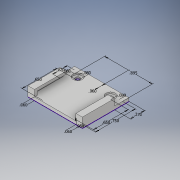
# Autodesk Inventor part: ShockSensorMount
Saved by Autodesk Inventor 2017 (Build 210142000, 142)
## iProperties
Created: 2018-12-12
Part Number: ShockSensorMount
Material: Glass
Document SubType Name: Modeling
Designer: S346795925
Density: 2.18 g/cm^3
Appearance: Clear
Author: S346795925
Autodesk Inventor part; units mm, degrees
sketch "Sketch1" plane through (0, 0, 0) normal (0, 1, 0) x (-1, 0, 0)
  line L0 (0, 0) -> (-25.781, 0)
  line L1 (-25.781, 0) -> (-25.781, -22.098)
  line L2 (-25.781, -22.098) -> (0, -22.098)
  line L3 (0, -22.098) -> (0, 0)
  line L4 (-1.524, -20.574) -> (-24.257, -20.574)
  line L5 (-24.257, -20.574) -> (-24.257, -1.524)
  line L6 (-24.257, -1.524) -> (-1.524, -1.524)
  line L7 (-1.524, -1.524) -> (-1.524, -20.574)
  line L8 (-3.048, 0) -> (-3.048, -1.524)
  line L9 (-22.733, 0) -> (-22.733, -1.524)
  line L10 (-3.048, -20.574) -> (-3.048, -22.098)
  line L11 (-3.048, -1.524) -> (-3.048, -20.574)
  line L12 (-22.733, -1.524) -> (-22.733, -20.574)
  line L13 (-22.733, -20.574) -> (-22.733, -22.098)
  line L14 (0, -15.24) -> (-1.524, -15.24)
  line L15 (-24.257, -15.24) -> (-25.781, -15.24)
  line L16 (-1.524, -15.24) -> (-3.048, -15.24)
  line L17 (-24.257, -15.24) -> (-22.733, -15.24)
  circle A0 centre (-5.08, -18.542) radius 1.0668
  circle A1 centre (-20.701, -2.032) radius 1.0668
  circle A2 centre (-20.701, -18.542) radius 1.0668
  circle A3 centre (-5.08, -2.032) radius 1.0668
  dimension "d2" = 1.524
  dimension "d3" = 19.05
  dimension "d4" = 22.733
  dimension "d5" = 1.524
  dimension "d6" = 1.524
  dimension "d10" = 6.858
  dimension "d11" = 6.858
  dimension "d19" = 2.1336
  dimension "d22" = 2.032
  dimension "d23" = 2.032
  dimension "d24" = 2.032
  dimension "d25" = 16.51
  dimension "d26" = 16.51
  constraints: 36 end point, 14 point on line, 12 perpendicular, 4 centre point, 4 parallel, 3 equal radius, 2 vertical alignment, 1 horizontal, 1 horizontal alignment, 3 other
  measures "d2" distance between parallel lines of L2 L4
  measures "d3" distance of L4.end L5.end
  measures "d4" distance of L4.start L4.end
  measures "d5" distance between parallel lines of L7 L8
  measures "d6" distance between parallel lines of L5 L9
  measures "d10" distance between parallel lines of L2 L14
  measures "d11" distance between parallel lines of L2 L15
  measures "d19" diameter of A1
  measures "d22" distance from line of L4 A0.centre
  measures "d23" distance from line of L11 A0.centre
  measures "d24" distance from line of L12 A2.centre
  measures "d25" distance of A3.centre A0.centre
  measures "d26" distance of A1.centre A2.centre
extrude "Extrusion2" add sketch "Sketch1" along normal blind 3.302 contours L3 L14 L7 L6 L8 L0 | L9 L6 L5 L15 L1 L0
ref_plane "Work Plane1" through (0, 3.302, 0) normal (0, 1, 0) x (1, 0, 0)
ref_plane "Work Plane2" through (0, 4.572, 0) normal (0, 1, 0) x (1, 0, 0)
extrude "Extrusion3" add sketch "Sketch1" along normal up to surface (1.27 mm away) from surface at 3.302 contours L3 L14 L7 L6 L8 L0 | L9 L6 L5 L15 L1 L0 | L6 L7 L16 L11 | L12 L17 L5 L6
ref_plane "Work Plane3" through (0, 1.524, 0) normal (0, 1, 0) x (1, 0, 0)
sketch "Sketch2" plane through (0, 1.524, 0) normal (0, 1, 0) x (1, 0, 0)
  circle A0 centre (5.08, 18.542) radius 1.0668 projected
  circle A1 centre (20.701, 18.542) radius 1.0668
  circle A2 centre (20.701, 2.032) radius 1.0668
  circle A3 centre (5.08, 2.032) radius 1.0668 projected
  circle A4 centre (20.701, 2.032) radius 1.0668 projected
  circle A5 centre (20.701, 18.542) radius 1.0668 projected
  point P0 (0, 0)
  constraints: 2 centre point, 2 concentric
extrude "Extrusion7" add sketch "Sketch1" along normal blind 1.524 contours L8 L6 A3 A1 L9 L0 | L3 L2 L10 L4 L7 L14 | L11 L4 L12 L6 A1 A3 | L6 L7 L16 L11 | L7 L4 L11 L16 | L12 L17 L5 L6 | A3 L6 | L6 A3 | L2 L13 L4 L10 | L15 L5 L4 L13 L2 L1 | A1 L6 | L6 A1 | L12 L4 L5 L17
hole "Hole2" at (20.701, 1.524, -18.542) at (5.08, 1.524, -18.542) direction (0, -1, 0) diameter 0.4763 end through all counterbore diameter 4.445 counterbore depth 0.762
body "Solid1"
